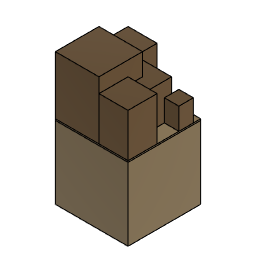
Stone cracking v4 (Autodesk Fusion 360 design; units mm, degrees)
Autodesk Fusion 360 part; units mm, degrees
sketch "Skizze1" plane through (0, 0, 0) normal (0, 0, 1) x (1, 0, 0)
  line L0 (0, 0) -> (50, 0) construction
  line L1 (50, 0) -> (50, 50)
  line L2 (50, 50) -> (0, 50)
  line L3 (0, 50) -> (0, 0) construction
  line L4 (0, 0) -> (30, 0)
  line L5 (30, 0) -> (30, 30)
  line L6 (30, 30) -> (0, 30)
  line L7 (0, 30) -> (0, 0)
  line L8 (0, 50) -> (20, 50)
  line L9 (20, 50) -> (20, 30)
  line L10 (20, 30) -> (0, 30)
  line L11 (0, 30) -> (0, 50)
  line L12 (50, 0) -> (30, 0)
  line L13 (30, 0) -> (30, 20)
  line L14 (30, 20) -> (50, 20)
  line L15 (50, 20) -> (50, 0)
  line L16 (20, 40) -> (40, 40)
  line L17 (40, 40) -> (40, 20)
  line L18 (20, 50) -> (30, 50)
  line L19 (30, 50) -> (30, 40)
  line L20 (30, 40) -> (20, 40)
  line L21 (20, 40) -> (20, 50)
  line L22 (40, 45) -> (50, 45)
  line L23 (50, 45) -> (50, 35)
  line L24 (50, 35) -> (40, 35)
  line L25 (40, 35) -> (40, 45)
  constraint horizontal L0
  constraint vertical L1
  constraint horizontal L2
  constraint vertical L3
  constraint coincident L0.start L3.end
  constraint horizontal L4
  constraint vertical L5
  constraint horizontal L6
  constraint vertical L7
  constraint horizontal L8
  constraint vertical L9
  constraint horizontal L10
  constraint vertical L11
  constraint coincident L6 L9.end
  constraint horizontal L12
  constraint vertical L13
  constraint horizontal L14
  constraint vertical L15
  constraint collinear L5 L13
  constraint perpendicular L5 L16
  constraint perpendicular L16 L17
  constraint horizontal L18
  constraint vertical L19
  constraint horizontal L20
  constraint vertical L21
  constraint midpoint L16 L19.end
  constraint horizontal L22
  constraint vertical L23
  constraint horizontal L24
  constraint vertical L25
  constraint coincident L1 L23.end
extrude "Extrusion1" add sketch "Skizze1" along normal blind 40 contours L4 L5 L6 L7 L10 L13 makes body 1 in component "Großer Block"
extrude "Extrusion1'" add sketch "Skizze1" along normal blind 30 separate body contours L1 L5 L12 L13 L14 L15 makes body 2 in component "Medium Block 1"
extrude "Extrusion1''" add sketch "Skizze1" along normal blind 30 separate body contours L2 L6 L8 L9 L10 L11 L21 makes body 3 in component "Medium Block 2#"
extrude "Extrusion1'''" add sketch "Skizze1" along normal blind 25 separate body contours L5 L6 L9 L14 L16 L17 L20 L25 makes body 4 in component "L Block"
extrude "Extrusion1''''" add sketch "Skizze1" along normal blind 15 separate body contours L2 L9 L16 L18 L19 L20 L21 makes body 5 in component "Smal Block 1"
extrude "Extrusion1'''''" add sketch "Skizze1" along normal blind 15 separate body contours L1 L17 L22 L23 L24 L25 makes body 6 in component "Smal Block 2"
extrude "Extrusion1''''''" add sketch "Skizze1" against normal blind 1 separate body makes body 7 in component "Ground"
extrude "Extrusion1'''''''" add 1 faces at (20, 26.6667, -1) along direction (0, 0, -1) blind 50 separate body on bodies 7 makes body 8 in component "Ground below"
component "Großer Block" placed x (1, 0, 0) y (0, 1, 0) z (0, 0, 1) at (0, 0, 0)
component "Medium Block 1" placed x (1, 0, 0) y (0, 1, 0) z (0, 0, 1) at (0, 0, 0)
component "Medium Block 2#" placed x (1, 0, 0) y (0, 1, 0) z (0, 0, 1) at (0, 0, 0)
component "L Block" placed x (1, 0, 0) y (0, 1, 0) z (0, 0, 1) at (0, 0, 0)
component "Smal Block 1" placed x (1, 0, 0) y (0, 1, 0) z (0, 0, 1) at (0, 0, 0)
component "Smal Block 2" placed x (1, 0, 0) y (0, 1, 0) z (0, 0, 1) at (0, 0, 0)
component "Ground" placed x (1, 0, 0) y (0, 1, 0) z (0, 0, 1) at (0, 0, 0)
component "Ground below" placed x (1, 0, 0) y (0, 1, 0) z (0, 0, 1) at (0, 0, 0)
